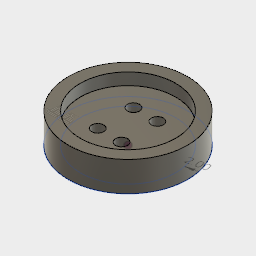
纽扣 v6 (Autodesk Fusion 360 design; units mm, degrees)
Autodesk Fusion 360 part; units mm, degrees
sketch "草图1" plane through (0, 0, 0) normal (0, 1, 0) x (1, 0, 0)
  circle A0 centre (0, 0) radius 10
  circle A1 centre (0, 0) radius 8
  dimension "d1" = 2
extrude "拉伸1" add sketch "草图1" along normal blind 3 contours A1 makes body 1
extrude "拉伸2" add sketch "草图1" along normal blind 5 separate body makes body 2
extrude "拉伸3" add sketch "草图1" along normal blind 5 separate body makes body 3
cylinder "圆柱体基本要素1" add diameter 2 height 20 placed x (1, 0, 0) y (0, 0, -1) z (0, 1, 0) at (14, 0, 13) separate body makes body 4
move_face "MoveFace1" to x (1, 0, 0) y (0, 1, 0) z (0, 0, 1) at (-15.9494, 0, -11.5593) 1 faces at (14.995, 13.3333, 13.0996) on bodies 4
move_face "MoveFace2" by (1.8042, 0.0218, -1.3256) 1 faces at (-1.2829, 20, 1.6689) on bodies 4
move_face "MoveFace3" to x (1, 0, 0) y (0, 1, 0) z (0, 0, 1) at (4.3904, -4.0318, -0.2923) 1 faces at (-0.9543, 13.3478, 1.5403) on bodies 4
move_body "移动1" bodies 4 to x (1, 0, 0) y (0, 1, 0) z (0, 0, 1) at (-1.8927, 0.1305, -1.2124)
move_body "移动2" bodies 4 to x (1, 0, 0) y (0, 1, 0) z (0, 0, 1) at (-0.1154, 0, 0.2949)
pattern_linear "R-阵列1" count 2 spacing 6 along (0, 0, 1) count 2 spacing 4 along (-1, 0, 0) of bodies 4 makes body 5 at (1.4279, 13.4783, 6.3304) makes body 6 at (-2.5684, 6.8044, 0.2807) makes body 7 at (-2.5684, 6.8044, 6.2807)
move_body "移动3" bodies 4 5 6 7 to x (1, 0, 0) y (0, 1, 0) z (0, 0, 1) at (1.5735, 0, -3.1469)
combine "合并1" operation cut target body 1 tool bodies 5 6 7 4
